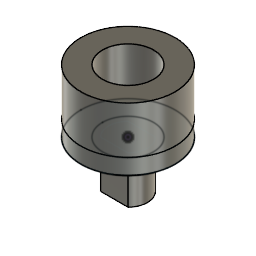
dctowheelmay25 (Autodesk Fusion 360 design; units mm, degrees)
Autodesk Fusion 360 part; units mm, degrees
sketch "Sketch1" plane through (0, 0, 0) normal (0, 0, 1) x (1, 0, 0)
  line L0 (1.75, -1.75) -> (-1.75, -1.75)
  line L1 (-1.75, -1.75) -> (-1.75, 1.75)
  line L2 (-1.75, 1.75) -> (1.75, 1.75)
  line L3 (1.75, 1.75) -> (1.75, -1.75)
  line L4 (1.75, -1.75) -> (-1.75, 1.75) construction
  line L5 (-1.75, -1.75) -> (1.75, 1.75) construction
  arc A0 (-1.75, 1.75) -> (-1.75, -1.75) centre (0, 0) ccw
  arc A1 (1.75, -1.75) -> (1.75, 1.75) centre (0, 0) ccw
  dimension "d1" = 3.5
  dimension "d2" = 3.5
  constraint horizontal L0
  constraint perpendicular L0 L1
  constraint parallel L0 L2
  constraint parallel L1 L3
  constraint coincident L4 A0.centre
  constraint coincident L5 A0.centre
  constraint coincident A0.centre A1.centre
  measures "d1" distance of L1.end L2.end
  measures "d2" distance of L0.end L1.end
extrude "Extrude1" add sketch "Sketch1" along normal blind 6 makes body 1
sketch "Sketch2" plane through (0, 0, 6) normal (0, 0, 1) x (-1, 0, 0)
  arc A0 (1.75, -1.75) -> (1.75, 1.75) centre (0, 0) ccw
  line L0 (1.75, 1.75) -> (-1.75, 1.75)
  arc A1 (-1.75, 1.75) -> (-1.75, -1.75) centre (0, 0) ccw
  line L1 (-1.75, -1.75) -> (1.75, -1.75)
  circle A2 centre (0, 0) radius 6
  circle A3 centre (0, 0) radius 3.25
  dimension "d5" = 12
  dimension "d6" = 6.5
  constraint coincident A0.centre A1.centre
  constraint concentric A2 A3
  measures "d5" diameter of A2
  measures "d6" diameter of A3
extrude "Extrude2" add sketch "Sketch2" along normal blind 2 contours A0 L0 A1 L1 | A2 | A3 bodies 1
extrude "Extrude3" add sketch "Sketch2" along normal blind 8 separate body contours A2 makes body 2
